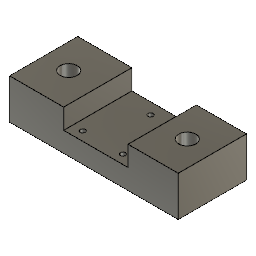
camera-mount v1 (Autodesk Fusion 360 design; units mm, degrees)
Autodesk Fusion 360 part; units mm, degrees
sketch "Sketch1" plane through (0, 0, 0) normal (0, 0, 1) x (1, 0, 0)
  line L0 (0, 0) -> (30, 0)
  line L1 (30, 0) -> (30, 30)
  line L2 (30, 30) -> (0, 30)
  line L3 (0, 30) -> (0, 0)
  circle A0 centre (5, 2.5) radius 1.25
  circle A1 centre (25, 2.5) radius 1.25
  circle A2 centre (15, 26.25) radius 1.25
  line L4 (-2, -2) -> (32, -2)
  line L5 (32, -2) -> (32, 32)
  line L6 (32, 32) -> (-2, 32)
  line L7 (-2, 32) -> (-2, -2)
  line L8 (-2, 32) -> (-27, 32)
  line L9 (-27, 32) -> (-27, -2)
  line L10 (-27, -2) -> (-2, -2)
  line L11 (-2, -2) -> (-2, 32)
  line L12 (32, 32) -> (57, 32)
  line L13 (57, 32) -> (57, -2)
  line L14 (57, -2) -> (32, -2)
  line L15 (32, -2) -> (32, 32)
  circle A3 centre (-14.5, 15) radius 4.25
  circle A4 centre (44.5, 15) radius 4.25
  dimension "d1" = 2.5
  dimension "d2" = 2.5
  dimension "d3" = 5
  dimension "d4" = 2.5
  dimension "d5" = 5
  dimension "d6" = 2.5
  dimension "d7" = 2.5
  dimension "d8" = 15
  dimension "d9" = 3.75
  dimension "d10" = 2
  dimension "d11" = 8.5
  dimension "d12" = 12.5
  dimension "d13" = 17
  dimension "d14" = 8.5
  dimension "d15" = 17
  dimension "d16" = 12.5
  constraint horizontal L0
  constraint vertical L1
  constraint horizontal L2
  constraint vertical L3
  constraint coincident L0.start L3.end
  constraint horizontal L8
  constraint vertical L9
  constraint horizontal L10
  constraint vertical L11
  constraint horizontal L12
  constraint vertical L13
  constraint horizontal L14
  constraint vertical L15
  measures "d1" diameter of A0
  measures "d2" distance of L0 A0.centre
  measures "d3" distance of L3 A0.centre
  measures "d4" diameter of A1
  measures "d5" distance of L1 A1.centre
  measures "d6" distance of L0 A1.centre
  measures "d7" diameter of A2
  measures "d8" distance of L3 A2.centre
  measures "d9" distance of L2 A2.centre
  measures "d11" diameter of A3
  measures "d12" distance of L9 A3.centre
  measures "d13" distance of L8 A3.centre
  measures "d14" diameter of A4
  measures "d15" distance of L12 A4.centre
  measures "d16" distance of L13 A4.centre
extrude "Extrude1" add sketch "Sketch1" along normal blind 10 contours L0 L1 L2 L3 | L4 L5 L6 L7 L11 L15 | L7 L8 L9 L10 L11 | L5 L12 L13 L14 L15
sketch "Sketch2" plane through (0, 0, 10) normal (0, 0, 1) x (-1, 0, 0)
  circle A0 centre (-5, -2.5) radius 1.25
  circle A1 centre (-44.5, -15) radius 4.25
  circle A2 centre (14.5, -15) radius 4.25
  circle A3 centre (-15, -26.25) radius 1.25
  circle A4 centre (-25, -2.5) radius 1.25
  line L0 (-57, -32) -> (27, -32)
  line L1 (27, -32) -> (27, 2)
  line L2 (27, 2) -> (-57, 2)
  line L3 (-57, 2) -> (-57, -32)
  line L4 (27, -32) -> (0, -32)
  line L5 (0, -32) -> (0, 2)
  line L6 (0, 2) -> (27, 2)
  line L7 (27, 2) -> (27, -32)
  line L8 (27, -32) -> (0, -32)
  line L9 (0, -32) -> (0, 2)
  line L10 (0, 2) -> (27, 2)
  line L11 (27, 2) -> (27, -32)
  constraint horizontal L4
  constraint vertical L5
  constraint horizontal L6
  constraint vertical L7
  constraint coincident L2 L5.end
  constraint coincident L0.end L1.start
  constraint horizontal L8
  constraint vertical L9
  constraint horizontal L10
  constraint vertical L11
extrude "Extrude2" add sketch "Sketch2" along normal blind 10 contours L0 L1 L2 L4 L5 L6 L7 L8 L9 L10 L11
sketch "Sketch3" plane through (0, 0, 10) normal (0, 0, 1) x (-1, 0, 0)
  line L0 (0, -32) -> (0, 2)
  line L1 (0, 2) -> (-57, 2)
  line L2 (-57, 2) -> (-57, -32)
  line L3 (-57, -32) -> (0, -32)
  circle A0 centre (-25, -2.5) radius 1.25
  circle A1 centre (-15, -26.25) radius 1.25
  circle A2 centre (-44.5, -15) radius 4.25
  circle A3 centre (-5, -2.5) radius 1.25
  line L4 (-57, -32) -> (-32, -32)
  line L5 (-32, -32) -> (-32, 2)
  line L6 (-32, 2) -> (-57, 2)
  line L7 (-57, 2) -> (-57, -32)
  constraint horizontal L4
  constraint vertical L5
  constraint horizontal L6
  constraint vertical L7
  constraint coincident L1 L5.end
  constraint coincident L2.end L3.start
extrude "Extrude3" add sketch "Sketch3" along normal blind 10 contours L1 L2 L3 L4 L5 L6 L7
